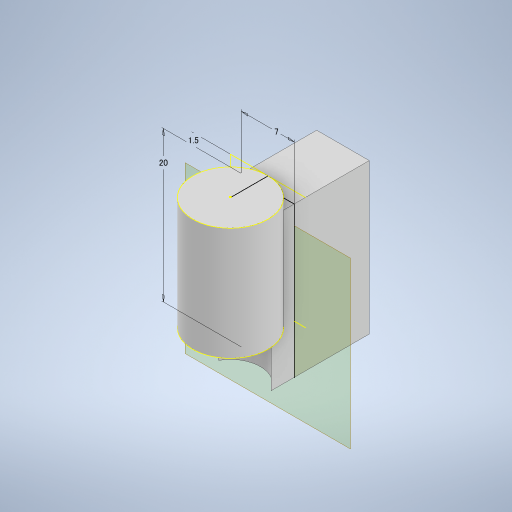
# Autodesk Inventor part: tale outer
Saved by Autodesk Inventor 2023 (Build 270158000, 158)
## iProperties
Created: 2022-10-23
Part Number: tale outer
Material: 一般
Document SubType Name: Modeling
Designer: ellie
Density: 1 g/cm^3
Appearance: 既定
Author: ellie
Autodesk Inventor part; units mm, degrees
ref_plane "YZ Plane" through (0, 0, 0) normal (1, 0, 0) x (0, 1, 0)
ref_plane "XZ Plane" through (0, 0, 0) normal (0, 1, 0) x (-1, 0, 0)
ref_plane "XY Plane" through (0, 0, 0) normal (0, 0, 1) x (1, 0, 0)
sketch "スケッチ1" plane through (0, 0, 0) normal (0, 1, 0) x (-1, 0, 0)
  circle A0 centre (0, 0) radius 5
  dimension "d0" = 10
  constraints: 1 centre point, 1 coincident
  measures "d0" diameter of A0
extrude "押し出し1" add sketch "スケッチ1" along normal blind 15
sketch "スケッチ2" plane through (0, 15, 0) normal (0, 1, 0) x (1, 0, 0)
  line L0 (0, 0) -> (0, 5)
  circle A0 centre (0, 0) radius 5 projected
  constraints: 2 end point, 1 vertical, 1 vertical alignment, 1 other
sketch "スケッチ3" plane through (0, 15, 0) normal (0, 1, 0) x (1, 0, 0)
  point P0 (0, 0)
sketch "スケッチ4" plane through (0, 0, 0) normal (0, -1, 0) x (1, 0, 0)
  line L0 (0, 0) -> (0, -5)
  circle A0 centre (0, 0) radius 5 projected
  constraints: 2 end point, 1 vertical, 1 vertical alignment, 1 other
ref_plane "作業平面1" through (0, 0, -5) normal (0, 0, -1) x (-1, 0, 0)
sketch "スケッチ5" plane through (0, 0, -5) normal (0, 0, -1) x (-1, 0, 0)
  line L0 (5, 15) -> (-5, 15) projected
  line L1 (0, 15) -> (0, 0)
  constraints: 2 end point, 1 midpoint, 1 vertical
sketch "スケッチ7" plane through (0, 0, 0) normal (0, -1, 0) x (1, 0, 0)
  circle A0 centre (0, 0) radius 4
  dimension "d3" = 8
  constraints: 1 centre point, 1 coincident
  measures "d3" diameter of A0
sketch "スケッチ8" plane through (0, 0, -5) normal (0, 0, -1) x (-1, 0, 0)
  line L0 (3.5, 13.5) -> (-3.5, 13.5)
  line L1 (-3.5, 13.5) -> (-3.5, -6.5)
  line L2 (-3.5, -6.5) -> (3.5, -6.5)
  line L3 (3.5, -6.5) -> (3.5, 13.5)
  line L4 (5, 15) -> (-5, 15) projected
  line L5 (0, 15) -> (0, 0) projected
  line L6 (5, 0) -> (5, 15) projected
  line L7 (5, 15) -> (-5, 15) projected
  line L8 (5, 0) -> (-5, 0) projected
  dimension "d6" = 1.5
  dimension "d7" = 7
  dimension "d8" = 20
  constraints: 8 end point, 2 parallel, 1 horizontal, 1 perpendicular, 1 other
  measures "d6" distance between parallel lines of L0 L4
  measures "d7" distance between parallel lines of L1 L3
  measures "d8" distance of L2.end L0.start
extrude "押し出し4" add sketch "スケッチ8" against normal blind 5 contours L3 L8 L5 L0 | L5 L8 L1 L0 | L3 L2 L1 L8
extrude "押し出し5" cut sketch "スケッチ7" along normal mid plane 26
extrude "押し出し6" add sketch "スケッチ8" along normal blind 10 contours L3 L8 L5 L0 | L5 L8 L1 L0 | L3 L2 L1 L8
